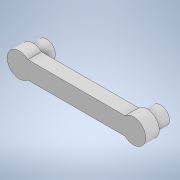
# Autodesk Inventor part: Component25
Saved by Autodesk Inventor 2022 (Build 260153000, 153)
## iProperties
Created: 2022-01-29
Part Number: Component25
Material: Generic
Document SubType Name: Modeling
Designer: Administrator
Density: 1 g/cm^3
Appearance: Default
Title: Component25
Author: Administrator
Autodesk Inventor part; units mm, degrees
ref_plane "YZ Plane" through (0, 0, 0) normal (1, 0, 0) x (0, 1, 0)
ref_plane "XZ Plane" through (0, 0, 0) normal (0, 1, 0) x (-1, 0, 0)
ref_plane "XY Plane" through (0, 0, 0) normal (0, 0, 1) x (1, 0, 0)
sketch "Sketch2" plane through (0, 0, 0) normal (0, 0, 1) x (1, 0, 0)
  circle A0 centre (-19.05, 0) radius 3.25
  line L0 (-15.9375, 3.25) -> (19.8375, 3.25)
  arc A1 (-15.9375, 3.25) -> (-15.9375, -3.25) centre (-19.05, 0) ccw
  arc A2 (19.8375, -3.25) -> (19.8375, 3.25) centre (22.95, 0) ccw
  circle A3 centre (22.95, 0) radius 3.25
  line L1 (-31.7023, 0) -> (39.7352, 0) construction
  line L2 (-15.9375, -3.25) -> (19.8375, -3.25)
  point P0 (0, 0)
  dimension "d4" = 6.5
  dimension "d6" = 9
  dimension "d7" = 6.5
  dimension "d8" = 42
  constraints: 6 end point, 4 centre point, 4 point on circle, 3 point on line, 2 coincident, 2 equal radius, 2 horizontal, 1 parallel, 1 symmetric about line
  measures "d4" diameter of A0
  measures "d6" diameter of A1
  measures "d7" distance between parallel lines of L2 L0
  measures "d8" distance of A2.centre A0.centre
extrude "Extrusion1" add sketch "Sketch2" along normal blind 5 contours A0 | L0 A2 L2 A1 | A3
extrude "Extrusion2" add sketch "Sketch2" against normal blind 5 contours A0 | A3
equation "\"d4\" = R"
equation "\"d6\" = R1"
equation "\"d7\" = width"
equation "\"d0\" = thickness"
equation "\"d2\" = thickness"
equation "\"R\" = 6.5"
equation "\"thickness\" = 5"
equation "\"width\" = 6.5"
equation "\"R1\" = 9"
body "Solid2"
